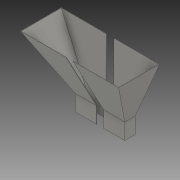
# Autodesk Inventor part: GearHopper
Saved by Autodesk Inventor 2016 (Build 200138000, 138)
## iProperties
Created: 2017-01-08
Part Number: GearHopper
Material: Generic
Document SubType Name: Modeling
Designer: hamblettk
Density: 1 g/cm^3
Appearance: Default
Author: hamblettk
Autodesk Inventor part; units mm, degrees
ref_plane "YZ Plane" through (0, 0, 0) normal (1, 0, 0) x (0, 1, 0)
ref_plane "XZ Plane" through (0, 0, 0) normal (0, 1, 0) x (-1, 0, 0)
ref_plane "XY Plane" through (0, 0, 0) normal (0, 0, 1) x (1, 0, 0)
sketch "Sketch33" plane through (0, 0, 0) normal (0, 0, 1) x (1, 0, 0)
  line L0 (0, 0) -> (63.5, 0)
  line L1 (0, 0) -> (0, 355.6)
  line L2 (0, 355.6) -> (254, 355.6)
  line L3 (254, 355.6) -> (63.5, 0)
  dimension "d86" = 63.5
  dimension "d87" = 355.6
  dimension "d88" = 254
  constraints: 8 end point, 1 horizontal, 1 perpendicular, 1 vertical
  measures "d86" distance of L0.start L0.end
  measures "d87" distance of L0.start L1.end
  measures "d88" distance of L1.end L2.end
extrude "Extrusion22" add sketch "Sketch33" along normal blind 609.6
sketch "Sketch34" plane through (0, 0, 0) normal (-1, 0, 0) x (0, 0, 1)
  line L0 (0, 0) -> (152.4, 0)
  line L1 (0, 0) -> (609.6, 0) projected
  line L2 (609.6, 0) -> (457.2, 0)
  line L3 (609.6, 0) -> (609.6, 355.6) projected
  line L4 (457.2, 0) -> (609.6, 355.6)
  line L5 (609.6, 355.6) -> (609.6, 0)
  line L6 (0, 0) -> (0, 355.6) projected
  line L7 (152.4, 0) -> (0, 355.6)
  line L8 (0, 355.6) -> (0, 0)
  dimension "d91" = 152.4
  dimension "d92" = 152.4
  constraints: 12 end point, 2 collinear, 2 point on line
  measures "d91" distance of L0.start L0.end
  measures "d92" distance of L1.end L2.end
extrude "Extrusion23" cut sketch "Sketch34" against normal blind 609.6
sketch "Sketch35" plane through (0, 0, 152.4) normal (0, -1, 0) x (1, 0, 0)
  line L0 (63.5, 0) -> (63.5, 304.8) projected
  line L1 (0, 0) -> (63.5, 0) projected
  line L2 (63.5, 0) -> (63.5, 304.8) projected
  line L3 (63.5, 304.8) -> (0, 304.8) projected
  line L4 (0, 0) -> (0, 304.8) projected
  point P0 (0, -152.4)
extrude "Extrusion24" add sketch "Sketch35" along normal blind 101.6
shell "Shell5" thickness 2.54 removed faces 1 at (169.3333, 355.6, 203.2)
sketch "Sketch36" plane through (0, -101.6, 152.4) normal (0, -1, 0) x (1, 0, 0)
  line L0 (0, 0) -> (63.5, 0) projected
  line L1 (63.5, 0) -> (63.5, 304.8) projected
  line L2 (63.5, 304.8) -> (0, 304.8) projected
  line L3 (0, 304.8) -> (0, 0) projected
  point P0 (0, -152.4)
extrude "Extrusion25" cut sketch "Sketch36" against normal blind 2.54
sketch "Sketch37" plane through (254, 355.6, 609.6) normal (0.88148, -0.4722214, 0) x (0, 0, -1)
  line L0 (606.8366, -1.3607) -> (2.7634, -1.3607) projected
  line L1 (2.7634, -1.3607) -> (282.1634, -1.3607)
  line L2 (606.8366, -1.3607) -> (327.4366, -1.3607)
  line L3 (282.1634, -1.3607) -> (327.4366, -1.3607)
  line L4 (327.4366, -1.3607) -> (327.4366, -405.0488)
  line L5 (327.4366, -405.0488) -> (282.1634, -405.0488)
  line L6 (282.1634, -405.0488) -> (282.1634, -1.3607)
  point P0 (609.6, -433.3985)
  dimension "d100" = 279.4
  dimension "d101" = 279.4
  constraints: 12 end point, 2 perpendicular, 2 point on line, 1 collinear, 1 vertical
  measures "d100" distance of L0.end L1.end
  measures "d101" distance of L0.start L2.end
extrude "Extrusion26" cut sketch "Sketch37" against normal blind 2.54
sketch "Sketch38" plane through (254, 355.6, 609.6) normal (0.88148, -0.4722214, 0) x (0, 0, -1)
  line L0 (282.1634, -1.3607) -> (327.4366, -1.3607) projected
  line L1 (282.1634, -1.3607) -> (282.1634, 0)
  line L2 (609.6, 0) -> (0, 0) projected
  line L3 (282.1634, 0) -> (327.4366, 0)
  line L4 (606.8366, -1.3607) -> (327.4366, -1.3607) projected
  line L5 (327.4366, 0) -> (327.4366, -1.3607)
  line L6 (327.4366, -1.3607) -> (282.1634, -1.3607)
  point P0 (609.6, -433.3985)
  constraints: 8 end point, 2 point on line, 1 collinear, 1 perpendicular, 1 vertical
extrude "Extrusion27" cut sketch "Sketch38" against normal blind 2.54
sketch "Sketch39" plane through (63.5, -99.06, 152.4) normal (1, 0, 0) x (0, 0, -1)
  line L0 (-175.0366, 98.5644) -> (-129.7634, 98.5644) projected
  line L1 (-175.0366, 98.5644) -> (-175.0366, 0)
  line L2 (-304.8, 0) -> (0, 0) projected
  line L3 (-175.0366, 0) -> (-129.7634, 0)
  line L4 (-129.7634, 0) -> (-129.7634, 98.5644)
  point P0 (152.4, 99.06)
  constraints: 6 end point, 2 point on line, 2 vertical
extrude "Extrusion28" cut sketch "Sketch39" against normal blind 2.54
sketch "Sketch40" plane through (63.5, -99.06, 152.4) normal (1, 0, 0) x (0, 0, -1)
  line L0 (-129.7634, 99.06) -> (-175.0366, 99.06) projected
  line L1 (-175.0366, 0) -> (-175.0366, 98.5644) projected
  line L2 (-175.0366, 99.06) -> (-175.0366, 98.5644)
  line L3 (-129.7634, 98.5644) -> (-129.7634, 0) projected
  line L4 (-175.0366, 98.5644) -> (-129.7634, 98.5644)
  line L5 (0, 99.06) -> (-129.7634, 99.06) projected
  line L6 (-129.7634, 99.06) -> (-129.7634, 98.5644)
  line L7 (-129.7634, 454.66) -> (-129.7634, 99.06) projected
  line L8 (-129.7634, 99.06) -> (-175.0366, 99.06)
  line L9 (-175.0366, 99.06) -> (-175.0366, 454.66) projected
  point P0 (152.4, 99.06)
  constraints: 8 end point, 2 perpendicular, 1 collinear, 1 vertical
extrude "Extrusion29" cut sketch "Sketch40" against normal blind 2.54
sketch "Sketch41" plane through (0, 355.6, 0) normal (-1, 0, 0) x (0, 0, 1)
  line L0 (0, 0) -> (282.1634, 0) projected
  line L1 (282.1634, -355.6) -> (282.1634, -454.66) projected
  line L2 (282.1634, 0) -> (282.1634, -454.66)
  line L3 (457.2, -454.66) -> (327.4366, -454.66) projected
  line L4 (282.1634, -454.66) -> (327.4366, -454.66)
  line L5 (327.4366, 0) -> (327.4366, -354.9625) projected
  line L6 (327.4366, -454.66) -> (327.4366, 0)
  line L7 (327.4366, 0) -> (282.1634, 0)
  point P0 (0, -355.6)
  constraints: 8 end point, 3 collinear, 1 perpendicular
extrude "Extrusion30" cut sketch "Sketch41" against normal blind 2.54
body "Solid9"
